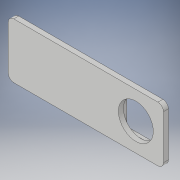
# Autodesk Inventor part: 30_Smartphone_Holder
Saved by Autodesk Inventor 2019 (Build 230136000, 136)
## iProperties
Created: 2019-07-16
Part Number: 30_Smartphone_Holder
Material: Generic
Document SubType Name: Modeling
Designer: marsikovabarbora
Density: 1 g/cm^3
Appearance: Default
Author: marsikovabarbora
Autodesk Inventor part; units mm, degrees
ref_plane "YZ Plane" through (0, 0, 0) normal (1, 0, 0) x (0, 1, 0)
ref_plane "XZ Plane" through (0, 0, 0) normal (0, 1, 0) x (-1, 0, 0)
ref_plane "XY Plane" through (0, 0, 0) normal (0, 0, 1) x (1, 0, 0)
sketch "Sketch1" plane through (0, 0, 0) normal (0, 0, 1) x (1, 0, 0)
  line L0 (-16.3829, -30.3318) -> (-62.1829, -30.3318)
  line L1 (-64.1829, -80.1318) -> (-14.3829, -80.1318) construction
  line L2 (35.6171, -80.1318) -> (-104.3829, -80.1318)
  line L3 (-104.3829, -80.1318) -> (-104.3829, -30.3318)
  line L4 (-104.3829, -30.3318) -> (35.6171, -30.3318)
  line L5 (35.6171, -30.3318) -> (35.6171, -80.1318)
  line L6 (-14.3829, -78.1318) -> (-14.3829, -32.3318)
  point P0 (-59.2829, -75.2318)
  point P1 (-19.2829, -75.2318)
  point P2 (-19.2829, -35.2318)
  point P3 (-59.2829, -35.2318)
extrude "Extrusion1" add sketch "Sketch1" along normal blind 4.5
sketch "Sketch4" plane through (0, 0, 4.5) normal (0, 0, 1) x (1, 0, 0)
  circle A0 centre (10.7171, -55.2318) radius 16.9 construction
  circle A1 centre (-9.2829, -35.2318) radius 1.45 projected
  circle A2 centre (30.7171, -35.2318) radius 1.45 projected
  arc A3 (-9.2829, -73.8318) -> (-9.2829, -76.6318) centre (-9.2829, -75.2318) ccw projected
  arc A4 (-9.2829, -73.8318) -> (-9.2829, -76.6318) centre (-9.2829, -75.2318) ccw projected
  arc A5 (30.7171, -76.6318) -> (30.7171, -73.8318) centre (30.7171, -75.2318) ccw projected
  circle A6 centre (10.7171, -55.2318) radius 15.75
  point P0 (0, 0)
  dimension "d48" = 31.5
  constraints: 1 centre point, 1 coincident
  measures "d48" diameter of A6
extrude "Extrusion3" cut sketch "Sketch4" against normal through all contours A6
sketch "Sketch3" plane through (0, 0, 4.5) normal (0, 0, 1) x (1, 0, 0)
  line L0 (-104.3829, -80.1318) -> (35.6171, -80.1318) projected
  line L1 (35.6171, -80.1318) -> (35.6171, -30.3318) projected
  line L2 (35.6171, -30.3318) -> (-104.3829, -30.3318) projected
  line L3 (-104.3829, -30.3318) -> (-104.3829, -80.1318) projected
  circle A0 centre (30.7171, -75.2318) radius 3
  circle A1 centre (-9.2829, -75.2318) radius 3
  circle A2 centre (-19.2829, -75.2318) radius 3
  circle A3 centre (-59.2829, -75.2318) radius 3
  circle A4 centre (30.7171, -35.2318) radius 3
  circle A5 centre (-9.2829, -35.2318) radius 3
  circle A6 centre (-19.2829, -35.2318) radius 3
  circle A7 centre (-59.2829, -35.2318) radius 3
  constraints: 8 centre point
extrude "Extrusion2" [suppressed]
fillet "Fillet1" radius 5 4 edges at (35.6171, -30.3318, 2.25) (-104.3829, -30.3318, 2.25) (-104.3829, -80.1318, 2.25) (35.6171, -80.1318, 2.25)
sketch "Sketch5" plane through (0, 0, 0) normal (0, 0, -1) x (-1, 0, 0)
  circle A0 centre (-10.7171, -55.2318) radius 15.75 construction
  arc A1 (-35.6171, -75.1318) -> (-30.6171, -80.1318) centre (-30.6171, -75.1318) ccw construction
  line L0 (-30.6171, -80.1318) -> (99.3829, -80.1318) construction
  arc A2 (99.3829, -80.1318) -> (104.3829, -75.1318) centre (99.3829, -75.1318) ccw construction
  line L1 (104.3829, -75.1318) -> (104.3829, -35.3318) construction
  arc A3 (104.3829, -35.3318) -> (99.3829, -30.3318) centre (99.3829, -35.3318) ccw construction
  line L2 (99.3829, -30.3318) -> (-30.6171, -30.3318) construction
  arc A4 (-30.6171, -30.3318) -> (-35.6171, -35.3318) centre (-30.6171, -35.3318) ccw construction
  line L3 (-35.6171, -35.3318) -> (-35.6171, -75.1318) construction
  line L4 (-27.5671, -72.0818) -> (6.1329, -72.0818) construction
  line L5 (6.1329, -72.0818) -> (6.1329, -38.3818) construction
  line L6 (6.1329, -38.3818) -> (-27.5671, -38.3818) construction
  line L7 (-27.5671, -38.3818) -> (-27.5671, -72.0818) construction
  line L8 (-27.5671, -72.0818) -> (6.1329, -38.3818) construction
  line L9 (6.1329, -72.0818) -> (-27.5671, -38.3818) construction
  line L10 (5.8829, -71.8318) -> (-27.3171, -71.8318)
  line L11 (-27.3171, -71.8318) -> (-27.3171, -38.6318)
  line L12 (-27.3171, -38.6318) -> (5.8829, -38.6318)
  line L13 (5.8829, -38.6318) -> (5.8829, -71.8318)
  line L14 (5.8829, -71.8318) -> (-27.3171, -38.6318) construction
  line L15 (-27.3171, -71.8318) -> (5.8829, -38.6318) construction
  line L16 (4.8829, -39.6318) -> (-26.3171, -39.6318)
  line L17 (-26.3171, -39.6318) -> (-26.3171, -70.8318)
  line L18 (-26.3171, -70.8318) -> (4.8829, -70.8318)
  line L19 (4.8829, -70.8318) -> (4.8829, -39.6318)
  point P0 (0, 0)
  dimension "d59" = 33.7
  dimension "d60" = 33.7
  dimension "d61" = 33.2
  dimension "d62" = 33.2
  dimension "d63" = 1
  constraints: 32 end point, 6 parallel, 4 midpoint, 3 perpendicular, 2 horizontal, 3 other
  measures "d59" distance of L6.end L5.end
  measures "d60" distance of L4.end L5.end
  measures "d61" distance of L11.end L12.end
  measures "d62" distance of L10.end L11.end
  measures "d63" distance between parallel lines of L12 L16
extrude "Extrusion4" add sketch "Sketch5" along normal blind 3
body "Solid1"
